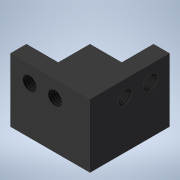
# Autodesk Inventor part: CONTOL_COMBI
Saved by Autodesk Inventor 2020 (Build 240168000, 168)
## iProperties
Created: 2020-06-03
Part Number: CONTOL_COMBI
Material: Generic
Document SubType Name: Modeling
Designer: Gebruiker
Density: 1 g/cm^3
Appearance: Default
Author: Gebruiker
Autodesk Inventor part; units mm, degrees
ref_plane "YZ Plane" through (0, 0, 0) normal (1, 0, 0) x (0, 1, 0)
ref_plane "XZ Plane" through (0, 0, 0) normal (0, 1, 0) x (-1, 0, 0)
ref_plane "XY Plane" through (0, 0, 0) normal (0, 0, 1) x (1, 0, 0)
sketch "Sketch1" plane through (0, 0, 0) normal (0, 0, 1) x (1, 0, 0)
  line L0 (-12.5, -10) -> (12.5, -10)
  line L1 (12.5, -10) -> (12.5, 10)
  line L2 (12.5, 10) -> (-12.5, 10)
  line L3 (-12.5, 10) -> (-12.5, -10)
  line L4 (-12.5, -10) -> (12.5, 10) construction
  line L5 (12.5, -10) -> (-12.5, 10) construction
  point P0 (0, 0)
  dimension "d0" = 25
  dimension "d1" = 20
  constraints: 12 end point, 2 midpoint, 2 parallel, 1 horizontal, 1 perpendicular
  measures "d0" distance of L2.end L1.end
  measures "d1" distance of L1.end L0.end
extrude "Extrusion1" add sketch "Sketch1" along normal blind 25
sketch "Sketch2" plane through (-12.5, 10, 0) normal (0, 1, 0) x (1, 0, 0)
  line L0 (0, 0) -> (25, 0) projected
  line L1 (0, 0) -> (20, 0)
  line L2 (20, 0) -> (20, -20)
  line L3 (20, -20) -> (0, -20)
  line L4 (0, -20) -> (0, 0)
  point P0 (12.5, 0)
  point P1 (20, 0)
  dimension "d4" = 20
  dimension "d5" = 20
  constraints: 8 end point, 2 parallel, 1 horizontal, 1 perpendicular
  measures "d4" distance of L2.end L3.end
  measures "d5" distance of L1.end L2.end
extrude "Extrusion2" cut sketch "Sketch2" against normal blind 10
sketch "Sketch3" plane through (7.5, 10, 0) normal (-1, 0, 0) x (0, 0, 1)
  circle A0 centre (6, -5) radius 2.25
  circle A1 centre (14, -5) radius 2.25
  line L0 (0, 0) -> (20, 0) projected
  line L1 (20, -10) -> (0, -10) projected
  line L2 (0, -10) -> (0, 0) projected
  line L3 (20, 0) -> (20, -10) projected
  dimension "d8" = 4.5
  dimension "d9" = 4.5
  dimension "d10" = 5
  dimension "d11" = 10
  dimension "d12" = 5
  dimension "d14" = 20
  dimension "d17" = 8
  dimension "d18" = 6
  constraints: 2 centre point
  measures "d8" diameter of A0
  measures "d9" diameter of A1
  measures "d10" distance from line of A0.centre L0
  measures "d11" distance between parallel lines of L1 L0
  measures "d12" distance from line of A1.centre L0
  measures "d14" distance between parallel lines of L3 L2
  measures "d17" distance of A1.centre A0.centre
  measures "d18" distance from line of L2 A0.centre
extrude "Extrusion3" cut sketch "Sketch3" against normal blind 5 contours A0 | A1
thread "Thread1" size "M4.5x0.75" class "6H" standard "ANSI Metric M Profile" length 100
thread "Thread2" size "M4.5x0.75" class "6H" standard "ANSI Metric M Profile" length 100
sketch "Sketch4" plane through (7.5, 10, 20) normal (0, 0, -1) x (-1, 0, 0)
  circle A0 centre (6, -5.25) radius 2.25
  circle A1 centre (14, -5.25) radius 2.25
  line L0 (0, 0) -> (20, 0) projected
  line L1 (20, 0) -> (20, -10) projected
  line L2 (0, 0) -> (0, -10) projected
  point P0 (7.5, -10)
  dimension "d25" = 4.5
  dimension "d26" = 4.5
  dimension "d27" = 8
  dimension "d28" = 3
  dimension "d29" = 3
  dimension "d30" = 6
  dimension "d31" = 6
  constraints: 2 centre point
  measures "d25" diameter of A0
  measures "d26" diameter of A1
  measures "d27" distance of A1.centre A0.centre
  measures "d28" distance edge to line of A1 L0
  measures "d29" distance edge to line of A0 L0
  measures "d30" distance from line of L1 A1.centre
  measures "d31" distance from line of L2 A0.centre
extrude "Extrusion4" cut sketch "Sketch4" against normal blind 5
thread "Thread3" size "M4.5x0.75" class "6H" standard "ANSI Metric M Profile" length 100
thread "Thread4" size "M4.5x0.75" class "6H" standard "ANSI Metric M Profile" length 100
body "Solid1"
